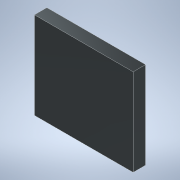
# Autodesk Inventor part: podpora silników
Saved by Autodesk Inventor 2022 (Build 260153000, 153)
## iProperties
Created: 2022-12-08
Part Number: podpora silników
Material: Iron, Cast
Document SubType Name: Modeling
Designer: Kamil
Density: 7.15 g/cm^3
Appearance: Iron Gray
Author: Kamil
Autodesk Inventor part; units mm, degrees
ref_plane "YZ Plane" through (0, 0, 0) normal (1, 0, 0) x (0, 1, 0)
ref_plane "XZ Plane" through (0, 0, 0) normal (0, 1, 0) x (-1, 0, 0)
ref_plane "XY Plane" through (0, 0, 0) normal (0, 0, 1) x (1, 0, 0)
sketch "Sketch1" plane through (0, 0, 0) normal (0, 0, 1) x (1, 0, 0)
  line L0 (-50, 48) -> (-50, -15.8) projected
  line L1 (-50, -15.8) -> (-18.25, -15.8) projected
  line L2 (-18.25, -15.8) -> (-18.25, -48) projected
  line L3 (-18.25, -48) -> (18.25, -48) projected
  line L4 (18.25, -48) -> (18.25, -15.8) projected
  line L5 (18.25, -15.8) -> (50, -15.8) projected
  line L6 (50, -15.8) -> (50, 48) projected
  line L7 (50, 48) -> (-50, 48) projected
  line L8 (18.25, -48) -> (-18.25, -48)
  line L9 (-18.25, -48) -> (-18.25, -15.8)
  line L10 (-18.25, -15.8) -> (18.25, -15.8)
  line L11 (18.25, -15.8) -> (18.25, -48)
  point P0 (0, 0)
  constraints: 8 end point, 2 parallel, 1 horizontal, 1 perpendicular
extrude "Extrusion1" add sketch "Sketch1" along normal blind 4.6 contours L10 L4 L3 L2
body "Solid1"
